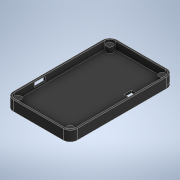
# Autodesk Inventor part: Основание
Saved by Autodesk Inventor 2022 (Build 260153000, 153)
## iProperties
Created: 2022-01-05
Part Number: Основание
Material: Каучук, силиконовый
Document SubType Name: Modeling
Designer: user
Density: 1.25 g/cm^3
Appearance: Резина — черная
Mass: 13.0261 g
Surface Area: 119.789 cm^2
Volume: 10.4209 cm^3
Author: user
Autodesk Inventor part; units mm, degrees
ref_plane "YZ Plane" through (0, 0, 0) normal (1, 0, 0) x (0, 1, 0)
ref_plane "XZ Plane" through (0, 0, 0) normal (0, 1, 0) x (-1, 0, 0)
ref_plane "XY Plane" through (0, 0, 0) normal (0, 0, 1) x (1, 0, 0)
sketch "Эскиз1" plane through (0, 0, 0) normal (0, 1, 0) x (-1, 0, 0)
  circle A0 centre (0, 0) radius 2.5
  circle A1 centre (0, -72.634) radius 2.5
  circle A2 centre (-41.385, -72.634) radius 2.5
  circle A3 centre (-41.385, 0) radius 2.5
  dimension "d1" = 5
  dimension "d3" = 5
  dimension "d5" = 5
  dimension "d7" = 5
  constraints: 4 centre point
  measures "d1" diameter of A0
  measures "d3" diameter of A1
  measures "d5" diameter of A2
  measures "d7" diameter of A3
extrude "Выдавливание1" add sketch "Эскиз1" against normal blind 4.5
sketch "Эскиз3" plane through (0, 0, 0) normal (0, 1, 0) x (1, 0, 0)
  line L0 (-4.5666, 0.8672) -> (-4.5666, 71.6657)
  line L1 (0.9251, 77.1637) -> (40.5431, 77.1677)
  line L2 (46.0198, 71.7001) -> (46.0348, 0.8657)
  line L3 (40.5334, -4.6343) -> (0.9348, -4.6343)
  arc A0 (-4.5666, 0.8672) -> (0.9348, -4.6343) centre (0.9348, 0.8672) ccw
  arc A1 (46.0198, 71.7001) -> (40.5431, 77.1677) centre (40.551, 71.699) ccw
  arc A2 (40.5334, -4.6343) -> (46.0348, 0.8657) centre (40.5319, 0.8687) ccw
  line L4 (35.1515, 48.9499) -> (35.1515, 54.3499)
  line L5 (35.1515, 54.6499) -> (35.1515, 48.6499)
  line L6 (35.4515, 54.6499) -> (40.8515, 54.6499)
  line L7 (41.1515, 54.6499) -> (35.1515, 54.6499)
  line L8 (40.8515, 48.6499) -> (35.4515, 48.6499)
  line L9 (41.1515, 54.3499) -> (41.1515, 48.9499)
  line L10 (41.1515, 48.6499) -> (41.1515, 54.6499)
  line L11 (35.1515, 48.6499) -> (41.1515, 48.6499)
  arc A3 (0.9251, 77.1637) -> (-4.5666, 71.6657) centre (1.3393, 71.2583) ccw
  constraints: 24 end point, 8 point on circle, 4 centre point, 3 tangent, 1 point on line
extrude "Выдавливание2" add sketch "Эскиз3" against normal blind 2 from surface at -4.5
sketch "Эскиз4" plane through (0.9348, -4.5, 4.6343) normal (0, 1, 0) x (1, 0, 0)
  line L0 (-5.5015, 5.5015) -> (-5.5015, 76.3) projected
  arc A0 (-4.2015, 5.5015) -> (0, 1.3) centre (0, 5.5015) ccw
  line L1 (45.085, 76.3344) -> (45.1, 5.5) projected
  line L2 (-0.0097, 81.798) -> (39.6083, 81.802) projected
  arc A1 (-0.0097, 80.5111) -> (-4.2035, 76.3214) centre (-0.0118, 76.3194) ccw
  arc A2 (43.785, 76.3344) -> (39.6083, 80.5111) centre (39.6083, 76.3344) ccw
  arc A3 (39.5985, 1.3) -> (43.785, 5.5) centre (39.585, 5.5) ccw
  line L3 (0, 1.3) -> (39.5985, 1.3)
  line L4 (43.785, 5.5) -> (43.785, 76.3344)
  line L5 (39.6083, 80.5111) -> (-0.0097, 80.5111)
  arc A4 (-5.5015, 5.5015) -> (0, 0) centre (0, 5.5015) ccw projected
  arc A5 (-0.0097, 81.798) -> (-5.5015, 76.3) centre (0.4044, 75.8926) ccw projected
  line L6 (-0.0097, 81.798) -> (39.6083, 81.802) projected
  arc A6 (45.085, 76.3344) -> (39.6083, 81.802) centre (39.6162, 76.3332) ccw projected
  arc A7 (39.5985, 0) -> (45.1, 5.5) centre (39.5971, 5.5029) ccw projected
  line L7 (39.5985, 0) -> (0, 0) projected
  arc A8 (-5.5015, 5.5015) -> (0, 0) centre (0, 5.5015) ccw
  arc A9 (-0.0097, 81.798) -> (-5.5015, 76.3) centre (0.4044, 75.8926) ccw
  arc A10 (45.085, 76.3344) -> (39.6083, 81.802) centre (39.6162, 76.3332) ccw projected
  arc A11 (45.085, 76.3344) -> (39.6083, 81.802) centre (39.6088, 76.3258) ccw
  arc A12 (39.5985, 0) -> (45.1, 5.5) centre (39.5971, 5.5029) ccw
  line L8 (-5.5015, 5.5015) -> (-5.5015, 76.3)
  line L9 (-0.0097, 81.798) -> (39.6083, 81.802)
  line L10 (45.085, 76.3344) -> (45.1, 5.5082)
  line L11 (39.5985, 0) -> (0, 0)
  line L12 (-4.2015, 5.5015) -> (-4.2035, 76.3214)
  circle A13 centre (40.4502, 77.2683) radius 1.5 projected
  point P0 (-0.9348, 4.6343)
  constraints: 17 point on circle, 16 end point, 8 centre point, 3 tangent, 2 horizontal, 1 collinear, 1 concentric, 1 perpendicular, 1 point on line
extrude "Выдавливание3" add sketch "Эскиз4" along normal blind 6 contours L0 A5 L2 A11 L1 A7 L7 A4 | A6 A11
sketch "Эскиз5" plane through (-4.5666, -6.5, -71.6657) normal (-1, 0, 0) x (0, 0, 1)
  line L0 (-5.498, 0) -> (0, 0) projected
  line L1 (55.3, 7) -> (55.3, 3.5)
  line L2 (-0.0344, 8) -> (70.8, 8) projected
  line L3 (76.3, 0) -> (76.3, 8) projected
  line L4 (46.8, 7) -> (46.8, 3.5)
  line L5 (46.8, 3.5) -> (55.3, 3.5)
  line L6 (-0.0344, 0) -> (70.8, 0) projected
  line L7 (46.8, 7) -> (55.3, 7)
  line L8 (74.1657, 6.5) -> (69.1657, 6.5) projected
  point P0 (71.6657, 6.5)
  point P1 (57.3, 6.5)
  dimension "d24" = 21
  dimension "d25" = 8.5
  dimension "d26" = 3.5
  constraints: 8 end point, 2 parallel, 2 vertical
  measures "d24" distance between parallel lines of L1 L3
  measures "d25" distance between parallel lines of L4 L1
  measures "d26" distance of L4.start L4.end
extrude "Выдавливание4" cut sketch "Эскиз5" against normal blind 6
